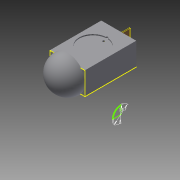
# Autodesk Inventor part: Pieza1
Saved by Autodesk Inventor 2013 (Build 170138000, 138)
## iProperties
Created: 2014-07-03
Part Number: Pieza1
Material: Genérico
Document SubType Name: Chapa
Designer: Administrador
Density: 1 g/cm^3
Sheet Metal Rule: Por defecto_mm
Author: Administrador
Autodesk Inventor part; units mm, degrees
ref_plane "YZ Plane" through (0, 0, 0) normal (1, 0, 0) x (0, 1, 0)
ref_plane "XZ Plane" through (0, 0, 0) normal (0, 1, 0) x (-1, 0, 0)
ref_plane "XY Plane" through (0, 0, 0) normal (0, 0, 1) x (1, 0, 0)
sketch "Boceto1" plane through (0, 0, 0) normal (0, 0, 1) x (1, 0, 0)
  line L0 (-17, 25) -> (17, 25)
  line L1 (17, 25) -> (17, -25)
  line L2 (17, -25) -> (-17, -25)
  line L3 (-17, -25) -> (-17, 25)
  line L4 (17, 25) -> (-17, -25) construction
  line L5 (-17, 25) -> (17, -25) construction
  point P0 (0, 0)
  point P1 (0, 0)
  dimension "d0" = 34
  dimension "d1" = 50
  constraints: 12 end point, 2 midpoint, 2 parallel, 1 coincident, 1 horizontal, 1 perpendicular
  measures "d0" distance of L1.end L2.end
  measures "d1" distance of L0.end L1.end
extrude "Extrusión1" add sketch "Boceto1" along normal mid plane 22
sketch "Boceto2" plane through (-17, -25, 11) normal (0, -1, 0) x (1, 0, 0)
  line L0 (34, 0) -> (34, -22) projected
  line L1 (0, 0) -> (34, 0) projected
  line L2 (0, 0) -> (0, -22) projected
  line L3 (34, -22) -> (0, -22) projected
  line L4 (32, 0) -> (0, -22) construction
  line L5 (0, 0) -> (32, -22) construction
  point P0 (17, -11)
  constraints: 4 end point
ref_plane "Plano de trabajo1" through (1, -25, 11) normal (1, 0, 0) x (0, 0, -1)
sketch "Boceto4" plane through (1, -25, 11) normal (1, 0, 0) x (0, 0, -1)
  arc A0 (62.0687, 50.9812) -> (70.5687, 42.4812) centre (70.5687, 50.9812) ccw
  arc A1 (63.0687, 50.9812) -> (70.5687, 43.4812) centre (70.5687, 50.9812) ccw
  line L0 (70.5687, 50.9812) -> (62.0687, 50.9812)
  line L1 (70.5687, 50.9812) -> (70.5687, 42.4812)
  point P0 (11, 25)
  dimension "d19" = 17
  dimension "d20" = 15
  constraints: 4 end point, 4 point on circle, 2 centre point, 2 point on line
  measures "d19" diameter of A0
  measures "d20" diameter of A1
ref_plane "Plano de trabajo2" through (0, -25, 11) normal (1, 0, 0) x (0, 0, -1)
sketch "Boceto5" plane through (0, -25, 11) normal (1, 0, 0) x (0, 0, -1)
  arc A0 (11, -16.622) -> (28, 0.378) centre (11, 0.378) ccw
  arc A1 (11, -14.622) -> (26, 0.378) centre (11, 0.378) ccw
  line L0 (11, 0.378) -> (11, -19.6766)
  line L1 (11, 0.378) -> (38.473, 0.378)
  point P0 (11, 25)
  dimension "d25" = 34
  dimension "d26" = 30
  constraints: 4 end point, 4 point on circle, 4 point on line, 2 centre point
  measures "d25" diameter of A0
  measures "d26" diameter of A1
revolve "Revolución2" add sketch "Boceto5" angle 360 about axis through (0, -24.622, 0) along (0, -1, 0) contours L0 A1 L1 A0
shell "Vaciado1" thickness 2 removed faces 1 at (5.6667, 25, 3.6667)
sketch "Boceto6" plane through (0, 0, -11) normal (0, 0, -1) x (-1, 0, 0)
  arc A0 (-0.9993, 13.463) -> (0.9993, 13.463) centre (0, 0) ccw
  arc A1 (0.9993, 13.463) -> (-0.9993, 13.463) centre (0, 13.4998) ccw
  dimension "d29" = 27
  dimension "d34" = 2
  constraints: 4 point on circle, 2 centre point
  measures "d29" diameter of A0
  measures "d34" diameter of A1
extrude "Extrusión2" cut sketch "Boceto6" against normal blind 1
sketch "Boceto7" plane through (0, 0, 11) normal (0, 0, 1) x (1, 0, 0)
  arc A0 (-0.9993, 13.463) -> (0.9993, 13.463) centre (0, 0) ccw projected
  arc A1 (0.9993, 13.463) -> (-0.9993, 13.463) centre (0, 13.4998) ccw projected
extrude "Extrusión3" cut sketch "Boceto7" against normal blind 1
hole "Hole2" at (0.5516, 9.7228, -10) direction (0, 0, 1) diameter 2 end through all
sketch "Boceto8" plane through (0, 0, -11) normal (0, 0, -1) x (-1, 0, 0)
  arc A0 (-0.9993, 13.463) -> (0.9993, 13.463) centre (0, 0) ccw projected
  arc A1 (0.9993, 13.463) -> (-0.9993, 13.463) centre (0, 13.4998) ccw projected
  arc A2 (-12.9615, -24.622) -> (-12.956, -25) centre (0, -24.622) ccw projected
  line L0 (-12.9615, -24.622) -> (-10.198, -24.622) projected
  arc A3 (-10.198, -24.622) -> (-10.191, -25) centre (0, -24.622) ccw projected
  line L1 (-10.191, -25) -> (10.191, -25) projected
  arc A4 (10.191, -25) -> (10.198, -24.622) centre (0, -24.622) ccw projected
  line L2 (10.198, -24.622) -> (12.9615, -24.622) projected
  arc A5 (12.956, -25) -> (12.9615, -24.622) centre (0, -24.622) ccw projected
  line L3 (12.956, -25) -> (17, -25) projected
  line L4 (17, -25) -> (17, 25) projected
  line L5 (17, 25) -> (-17, 25) projected
  line L6 (-17, 25) -> (-17, -25) projected
  line L7 (-17, -25) -> (-12.956, -25) projected
equation "\"Radio_pliegue\" = Grosor"
equation "\"Anchura_desahogo_plegado\" = Grosor"
equation "\"Profundidad_desahogo_plegado\" = 0.5 * Grosor"
equation "\"Tamaño_destalonado\" = 4 * Grosor"
equation "\"Remanente_mínimo\" = 2 * Grosor"
equation "\"Radiodetransición\" = Radio_pliegue"
equation "\"Tamaño_de_radio_de_Jacobi\" = Radio_pliegue"
equation "\"TamañoSeparación\" = Grosor"
equation "\"Grosor\" = 0.5"
